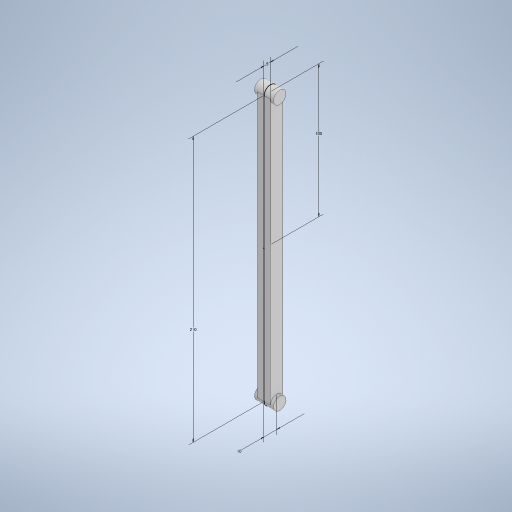
# Autodesk Inventor part: body
Saved by Autodesk Inventor 2024.3 (Build 283343000, 343)
## iProperties
Created: 2025-01-18
Part Number: body
Material: 一般
Document SubType Name: Modeling
Designer: yuu53
Density: 1 g/cm^3
Appearance: 既定
Author: yuu53
Autodesk Inventor part; units mm, degrees
ref_plane "YZ Plane" through (0, 0, 0) normal (1, 0, 0) x (0, 1, 0)
ref_plane "XZ Plane" through (0, 0, 0) normal (0, 1, 0) x (-1, 0, 0)
ref_plane "XY Plane" through (0, 0, 0) normal (0, 0, 1) x (1, 0, 0)
sketch "スケッチ1" plane through (0, 0, 0) normal (1, 0, 0) x (0, 1, 0)
  line L0 (-105, 5) -> (105, 5)
  line L1 (105, 5) -> (105, -5)
  line L2 (105, -5) -> (-105, -5)
  line L3 (-105, -5) -> (-105, 5)
  circle A0 centre (-105, 0) radius 5
  circle A1 centre (105, 0) radius 5
  point P0 (0, 0)
  point P1 (0, 5)
  dimension "d0" = 210
  dimension "d1" = 10
  dimension "d2" = 5
  dimension "d3" = 105
  constraints: 8 end point, 3 coincident, 3 midpoint, 2 parallel, 2 vertical alignment, 1 horizontal, 1 perpendicular, 4 other
  measures "d0" distance of L0.start L0.end
  measures "d1" distance of L2.end L0.start
  measures "d2" distance of point (0, 5) point (0, 0)
  measures "d3" distance of point (105, 0) point (0, 0)
extrude "押し出し1" add sketch "スケッチ1" along normal blind 5 and the other way blind 5 contours A0 L3 | L0 A1 L2 A0 | L1 A1 picked at (-103.4984, 0.7231) picked at (102.0793, -0.9468)
extrude "押し出し2" add sketch "スケッチ1" along normal blind 7.5 and the other way blind 7.5 contours A0 L3 | L3 A0 | A1 L1 | L1 A1
